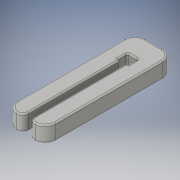
# Autodesk Inventor part: BaseClip
Saved by Autodesk Inventor 2016 (Build 200138000, 138)
## iProperties
Created: 2016-03-05
Part Number: BaseClip
Material: Generic
Document SubType Name: Modeling
Designer: yash
Density: 1 g/cm^3
Appearance: Default
Author: yash
Autodesk Inventor part; units mm, degrees
ref_plane "YZ Plane" through (0, 0, 0) normal (1, 0, 0) x (0, 1, 0)
ref_plane "XZ Plane" through (0, 0, 0) normal (0, 1, 0) x (-1, 0, 0)
ref_plane "XY Plane" through (0, 0, 0) normal (0, 0, 1) x (1, 0, 0)
sketch "Sketch1" plane through (0, 0, 0) normal (0, 1, 0) x (-1, 0, 0)
  line L0 (0, 0) -> (-4.7625, 0)
  line L1 (-4.7625, 0) -> (-4.7625, -28.575)
  line L2 (0, -1.7454) -> (0, 0)
  line L3 (-11.43, -1.7454) -> (-11.43, -38.1)
  line L4 (-11.43, -38.1) -> (0, -38.1)
  line L5 (0, -38.1) -> (0, -1.7454)
  line L6 (-6.6675, -28.575) -> (-6.6675, 0)
  line L7 (-6.6675, 0) -> (-11.43, 0)
  line L8 (-11.43, 0) -> (-11.43, -1.7454)
  line L9 (-4.1275, -31.75) -> (-7.3025, -31.75)
  line L10 (-7.3025, -31.75) -> (-7.3025, -28.575)
  line L11 (-4.1275, -28.575) -> (-4.1275, -31.75)
  line L12 (-7.3025, -28.575) -> (-6.6675, -28.575)
  line L13 (-4.7625, -28.575) -> (-4.1275, -28.575)
  point P0 (-5.715, -31.75)
  point P1 (-5.715, -38.1)
  dimension "d29" = 38.1
  dimension "d30" = 11.43
  dimension "d31" = 3.175
  dimension "d32" = 3.175
  dimension "d33" = 0.635
  dimension "d34" = 0.635
  dimension "d35" = 28.575
  dimension "d36" = 28.575
  dimension "d37" = 4.7625
  dimension "d38" = 1.7454
  constraints: 28 end point, 8 parallel, 2 equal length, 2 horizontal, 2 midpoint, 2 perpendicular, 1 vertical alignment
  measures "d29" distance between parallel lines of L4 L0
  measures "d30" distance of L3.end L4.end
  measures "d31" distance of L9.start L9.end
  measures "d32" distance of L9.end L10.end
  measures "d33" distance of L10.end L6.start
  measures "d34" distance of L1.end L11.start
  measures "d35" distance of L0.end L1.end
  measures "d36" distance of L6.start L6.end
  measures "d37" distance of L6.end L7.end
  measures "d38" distance of L2.start L0.start
extrude "Extrusion1" add sketch "Sketch1" along normal blind 4.7625
fillet "Fillet1" radius 3.175 4 edges at (0, 2.3813, -38.1) (11.43, 2.3813, -38.1) (0, 2.3813, 0) (11.43, 2.3813, 0)
fillet "Fillet2" radius 1.7272 2 edges at (6.6675, 2.3813, 0) (4.7625, 2.3813, 0)
fillet "Fillet3" radius 0.4318 20 edges at (10.5001, 4.7625, -37.1701) (5.715, 4.7625, -38.1) (0.9299, 4.7625, -37.1701) (0.8169, 4.7625, -1.0489) (4.1962, 4.7625, -0.4551) (4.7625, 4.7625, -15.1545) (10.6131, 4.7625, -1.0489) (7.2338, 4.7625, -0.4551) (6.6675, 4.7625, -15.1545) (11.43, 4.7625, -19.05) (10.5001, 0, -37.1701) (5.715, 0, -38.1) (0.9299, 0, -37.1701) (0.8169, 0, -1.0489) (4.1962, 0, -0.4551) (4.7625, 0, -15.1545) (10.6131, 0, -1.0489) (7.2338, 0, -0.4551) (6.6675, 0, -15.1545) (11.43, 0, -19.05)
fillet "Fillet4" radius 0.4318 8 edges at (4.1275, 4.7625, -30.1625) (7.3025, 4.7625, -30.1625) (5.715, 4.7625, -31.75) (4.1275, 0, -30.1625) (5.715, 0, -31.75) (7.3025, 0, -30.1625) (7.3025, 2.3813, -31.75) (4.1275, 2.3813, -31.75)
body "Solid1"
